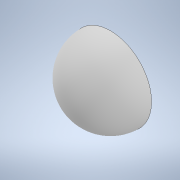
# Autodesk Inventor part: ball
Saved by Autodesk Inventor 2022 (Build 260153000, 153)
## iProperties
Created: 2022-11-11
Part Number: ball
Material: Generic
Document SubType Name: Modeling
Designer: trevo
Density: 1 g/cm^3
Appearance: Default
Author: trevo
Autodesk Inventor part; units mm, degrees
ref_plane "YZ Plane" through (0, 0, 0) normal (1, 0, 0) x (0, 1, 0)
ref_plane "XZ Plane" through (0, 0, 0) normal (0, 1, 0) x (-1, 0, 0)
ref_plane "XY Plane" through (0, 0, 0) normal (0, 0, 1) x (1, 0, 0)
sketch "Sketch1" plane through (0, 0, 0) normal (0, 0, 1) x (1, 0, 0)
  circle A0 centre (0, 0) radius 6.35
  line L0 (0, 6.35) -> (0, -6.35)
  dimension "d0" = 12.7
  constraints: 2 end point, 2 point on circle, 1 centre point, 1 coincident, 1 vertical
  measures "d0" diameter of A0
revolve "Revolution1" add sketch "Sketch1" angle 180 about axis through (0, 6.35, 0) along (0, 1, 0) picked at (-3.484, 2.1167) contours L0 A0
sketch "Sketch3" plane through (0, 0, 0) normal (0, 0, -1) x (-1, 0, 0)
  line L0 (0, 0) -> (0, 1.524) construction
  line L1 (0, 1.524) -> (1.524, 1.524) construction
  line L2 (0, 0) -> (0, -1.524) construction
  line L3 (0, -1.524) -> (-1.524, -1.524) construction
  line L4 (1.524, 1.524) -> (-1.524, 1.524)
  line L5 (-1.524, 1.524) -> (-1.524, -1.524)
  line L6 (-1.524, -1.524) -> (1.524, -1.524)
  line L7 (1.524, -1.524) -> (1.524, 1.524)
  dimension "d5" = 1.524
  dimension "d11" = 1.524
  dimension "d12" = 1.524
  dimension "d13" = 1.524
  constraints: 16 end point, 2 horizontal, 2 parallel, 2 perpendicular, 2 vertical
  measures "d5" distance of L0.start L0.end
  measures "d11" distance of L0.end L1.end
  measures "d12" distance of L0.start L2.end
  measures "d13" distance of L2.end L3.end
extrude "Extrusion3" cut sketch "Sketch3" against normal blind 5.08
body "Solid2"
